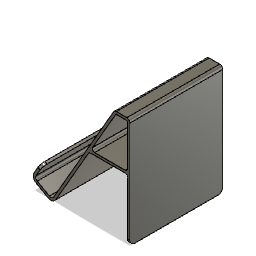
phone_stand (Autodesk Fusion 360 design; units mm, degrees)
Autodesk Fusion 360 part; units mm, degrees
sketch "Sketch1" plane through (0, 0, 0) normal (0, 0, 1) x (1, 0, 0)
  line L0 (-6.2583, 15.1603) -> (-10.2583, 8.2321)
  line L1 (-9.5263, 5.5) -> (-1.7321, 1)
  line L2 (1, 1.7321) -> (39.8372, 69)
  line L3 (41.5692, 70) -> (48.4145, 70)
  line L4 (50.4145, 68) -> (50.4145, -0.8679)
  line L5 (0, 0) -> (50.4145, 0) construction
  arc A0 (-10.2583, 8.2321) -> (-9.5263, 5.5) centre (-8.5263, 7.2321) ccw
  arc A1 (-1.7321, 1) -> (1, 1.7321) centre (-0.7321, 2.7321) ccw
  arc A2 (41.5692, 70) -> (39.8372, 69) centre (41.5692, 68) ccw
  arc A3 (50.4145, 68) -> (48.4145, 70) centre (48.4145, 68) ccw
  line L6 (-7.644, 15.9603) -> (-11.644, 9.0321)
  arc A4 (-11.644, 9.0321) -> (-10.3263, 4.1144) centre (-8.5263, 7.2321) ccw
  line L7 (-10.3263, 4.1144) -> (-2.5321, -0.3856)
  arc A5 (-2.5321, -0.3856) -> (2.3856, 0.9321) centre (-0.7321, 2.7321) ccw
  line L8 (2.3856, 0.9321) -> (41.2228, 68.2)
  arc A6 (41.5692, 68.4) -> (41.2228, 68.2) centre (41.5692, 68) ccw
  line L9 (41.5692, 68.4) -> (48.4145, 68.4)
  arc A7 (48.8145, 68) -> (48.4145, 68.4) centre (48.4145, 68) ccw
  line L10 (48.8145, 68) -> (48.8145, -0.8679)
  line L11 (-7.644, 15.9603) -> (-6.2583, 15.1603)
  line L12 (48.8145, -0.8679) -> (50.4145, -0.8679)
  line L13 (48.8145, -0.8679) -> (-0.7321, -0.8679) construction
  line L14 (48.8145, 38.4) -> (24.0178, 38.4)
  line L15 (48.8145, 40) -> (24.0178, 40)
  point P0 (-11.2583, 6.5)
  point P1 (40.4145, 70)
  point P2 (50.4145, 70)
  dimension "d1" = 10
  dimension "d2" = 90
  dimension "d3" = 13
  dimension "d4" = 90
  dimension "d5" = 10
  dimension "d6" = 60
  dimension "d7" = 70
  dimension "d8" = 2
  dimension "d9" = 1.6
  dimension "d12" = 1.6
  dimension "d13" = 30
  constraint coincident L5.start origin
  constraint horizontal L3
  constraint perpendicular L3 L4
  constraint coincident L4 L5.end
  constraint perpendicular L4 L5
  constraint coincident P0 L0
  constraint coincident P0 L1
  constraint tangent L0 A0
  constraint tangent L1 A0
  constraint coincident L5.start L1
  constraint coincident L5.start L2
  constraint tangent L1 A1
  constraint tangent L2 A1
  constraint equal A0 A1
  constraint coincident P1 L2
  constraint coincident P1 L3
  constraint tangent L2 A2
  constraint tangent L3 A2
  constraint equal A0 A2
  constraint coincident P2 L3
  constraint coincident P2 L4
  constraint tangent L3 A3
  constraint tangent L4 A3
  constraint equal A0 A3
  constraint perpendicular L0 L11
  constraint perpendicular L4 L12
  constraint coincident A5 L13.end
  constraint tangent A5 L13
  constraint horizontal L13
  constraint coincident L10 L14.start
  constraint coincident L8 L14.end
  constraint perpendicular L10 L14
  measures "d1" distance of L0.start P0
  measures "d2" angle of L0 L1
  measures "d3" distance of P0 L5.start
  measures "d4" angle of L1 L2
  measures "d5" distance of P1 P2
  measures "d6" angle of L2 L5
  measures "d7" distance of L3 L5
  measures "d8" radius of A0
  measures "d13" distance of L9 L14
extrude "Extrude1" add sketch "Sketch1" along normal mid plane 60 contours L0 L1 L2 L3 L4 A0 A1 A2 A3 L6 A4 L7 A5 L8 A6 L9 A7 L10 L11 L12 | L8 L10 L14 L15
fillet "Fillet1" radius 1.5 4 edges at (48.8145, 40, 0) (24.9415, 40, 0) (24.0178, 38.4, 0) (48.8145, 38.4, 0)
fillet "Fillet2" radius 3 4 edges at (-6.9512, 15.5603, 30) (-6.9512, 15.5603, -30) (49.6145, -0.8679, -30) (49.6145, -0.8679, 30)
